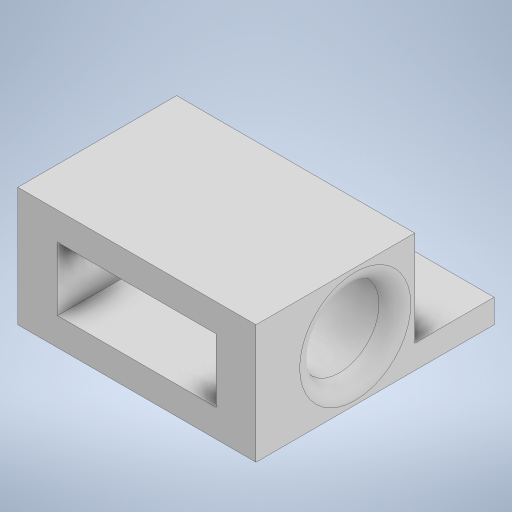
# Autodesk Inventor part: Pièce1
Saved by Autodesk Inventor 2024.1 (Build 281209000, 209)
## iProperties
Created: 2024-05-05
Part Number: Pièce1
Material: Générique
Document SubType Name: Modeling
Designer: chass
Density: 1 g/cm^3
Appearance: Par défaut
Author: chass
## iProperties of the stored document Pièce1_Impression 3D.ipt
Created: 2024-05-05
Part Number: Pièce1_Impression 3D
Material: Générique
Document SubType Name: Modeling
Designer: chass
Density: 1 g/cm^3
Appearance: Par défaut
Author: chass
Autodesk Inventor part; units mm, degrees
ref_plane "YZ Plane" through (0, 0, 0) normal (1, 0, 0) x (0, 1, 0)
ref_plane "XZ Plane" through (0, 0, 0) normal (0, 1, 0) x (-1, 0, 0)
ref_plane "XY Plane" through (0, 0, 0) normal (0, 0, 1) x (1, 0, 0)
sketch "Esquisse1" plane through (0, 0, 0) normal (1, 0, 0) x (0, 1, 0)
  circle A0 centre (0, 0) radius 5
  line L0 (7.5, 7.5) -> (-7.5, 7.5)
  line L1 (-7.5, 7.5) -> (-7.5, -7.5)
  line L2 (-7.5, -7.5) -> (7.5, -7.5)
  line L3 (7.5, -7.5) -> (7.5, 7.5)
  line L4 (7.5, 7.5) -> (-7.5, -7.5)
  line L5 (-7.5, 7.5) -> (7.5, -7.5)
  point P0 (0, 0)
  dimension "d0" = 10
  dimension "d1" = 15
  dimension "d2" = 15
  constraints: 12 end point, 2 coincident, 2 midpoint, 2 parallel, 1 centre point, 1 horizontal, 1 perpendicular
  measures "d0" diameter of A0
  measures "d1" distance of L1.end L2.end
  measures "d2" distance of L2.end L0.start
extrude "Extrusion1" add sketch "Esquisse1" along normal blind 30 contours A0 L4 L3 L5 | A0 L5 L0 L4 | L5 L2 L4 A0 | A0 L4 L1 L5
sketch "Esquisse6" plane through (0, -7.5, 7.5) normal (0, 0, 1) x (1, 0, 0)
  line L0 (0, 7.5) -> (30, 7.5)
  line L1 (30, 15) -> (30, 0) projected
  line L2 (5, 11.5) -> (25, 11.5)
  line L3 (25, 11.5) -> (25, 7.5)
  line L4 (25, 7.5) -> (5, 7.5)
  line L5 (5, 7.5) -> (5, 11.5)
  line L6 (0, 15) -> (0, 0) projected
  line L7 (0, 11.5) -> (5, 11.5)
  line L8 (5, 3.5) -> (25, 3.5)
  line L9 (25, 3.5) -> (25, 7.5)
  line L10 (5, 7.5) -> (5, 3.5)
  dimension "d14" = 4
  dimension "d15" = 5
  dimension "d16" = 20
  constraints: 18 end point, 2 parallel, 2 perpendicular, 2 point on line, 2 symmetric about line, 1 horizontal, 1 midpoint
  measures "d14" distance of L2.end L3.end
  measures "d15" distance of L7.start L2.start
  measures "d16" distance of L2.start L2.end
extrude "Extrusion5" cut sketch "Esquisse6" against normal blind 5 contours L5 L2 L3 L0 | L0 L9 L8 L10
sketch "Esquisse8" plane through (0, -7.5, 7.5) normal (0, 0, 1) x (1, 0, 0)
  line L0 (5, 11.5) -> (25, 11.5) projected
  line L1 (25, 3.5) -> (5, 3.5) projected
  line L2 (5, 11.5) -> (25, 11.5)
  line L3 (25, 11.5) -> (25, 3.5)
  line L4 (25, 3.5) -> (5, 3.5)
  line L5 (5, 3.5) -> (5, 11.5)
  line L6 (0, 15) -> (30, 15) projected
  line L7 (30, 15) -> (30, 0) projected
  line L8 (0, 15) -> (30, 15)
  line L9 (30, 15) -> (30, 0)
  line L10 (30, 0) -> (0, 0)
  line L11 (0, 0) -> (0, 15)
  point P0 (0, 7.5)
  constraints: 16 end point, 4 parallel, 2 horizontal, 2 perpendicular
extrude "Extrusion6" add sketch "Esquisse8" along normal blind 5
sketch "Esquisse9" plane through (0, -7.5, -7.5) normal (0, 0, -1) x (-1, 0, 0)
  line L0 (0, 0) -> (-30, 0) projected
  line L1 (-30, 0) -> (0, 0)
  line L2 (0, 0) -> (0, 3)
  line L3 (0, 3) -> (-30, 3)
  line L4 (-30, 3) -> (-30, 0)
  point P0 (0, 7.5)
  constraints: 8 end point, 2 parallel, 1 horizontal, 1 perpendicular
extrude "Extrusion7" add sketch "Esquisse9" along normal blind 10
sketch "Esquisse10" plane through (0, -4.5, -7.5) normal (0, 1, 0) x (1, 0, 0)
  circle A0 centre (15, 5) radius 1.75
  line L0 (0, 10) -> (30, 10) projected
  line L1 (30, 0) -> (30, 10) projected
  point P0 (0, -7.5)
  dimension "d23" = 3.5
  dimension "d24" = 5
  dimension "d25" = 15
  constraints: 1 centre point
  measures "d23" diameter of A0
  measures "d24" distance from line of L0 A0.centre
  measures "d25" distance from line of L1 A0.centre
extrude "Extrusion8" cut sketch "Esquisse10" against normal blind 10
fillet "Congé2" radius 2 2 edges at (0, -5, 0) (30, -5, 0)
